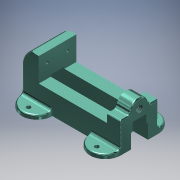
# Autodesk Inventor part: VS-001 (BASE)
Saved by Autodesk Inventor 2017 (Build 210142000, 142)
## iProperties
Created: 2016-11-28
Part Number: VS-001 (BASE)
Material: Iron, Cast
Document SubType Name: Modeling
Designer: OCCC
Mass: 2711.86 g
Surface Area: 697.582 cm^2
Volume: 379.281 cm^3
Density: 7.15 g/cm^3
Appearance: Machined 02
Author: OCCC
Autodesk Inventor part; units mm, degrees
ref_plane "YZ Plane" through (0, 0, 0) normal (1, 0, 0) x (0, 1, 0)
sketch "Sketch1" plane through (0, 0, 0) normal (0, 0, 1) x (1, 0, 0)
  line L0 (0, 0) -> (-184.15, 0)
  line L1 (-184.15, 0) -> (-184.15, 53.975)
  line L2 (-166.8312, 84.1375) -> (-152.4, 84.1375)
  line L3 (-152.4, 84.1375) -> (-152.4, 39.6875)
  line L4 (-152.4, 39.6875) -> (-25.4, 39.6875)
  line L5 (-25.4, 39.6875) -> (-25.4, 55.5625)
  line L6 (-25.4, 55.5625) -> (0, 55.5625)
  line L7 (0, 55.5625) -> (0, 0)
  line L8 (-184.15, 53.975) -> (-149.225, 53.975) construction
  arc A0 (-166.8312, 84.1375) -> (-184.15, 53.975) centre (-149.225, 53.975) ccw
  dimension "d0" = 184.15
  dimension "d1" = 55.5625
  dimension "d4" = 25.4
  dimension "d5" = 15.875
  dimension "d6" = 127
  dimension "d7" = 30.1625
  dimension "d8" = 34.925
  dimension "d9" = 84.1375
  constraints: 18 end point, 7 perpendicular, 2 horizontal, 2 point on circle, 1 centre point, 1 coincident
  measures "d0" distance of L0.start L0.end
  measures "d1" distance of L6.end L0.start
  measures "d4" distance of L5.end L6.end
  measures "d5" distance of L4.end L5.end
  measures "d6" distance of L3.end L4.end
  measures "d7" distance between parallel lines of L2 L8
  measures "d8" distance of L1.end L8.end
  measures "d9" distance between parallel lines of L0 L2
extrude "Extrusion1" add sketch "Sketch1" against normal blind 69.85
sketch "Sketch2" plane through (0, 0, 0) normal (0, 1, 0) x (-1, 0, 0)
  arc A0 (184.15, 0) -> (127, 0) centre (155.575, 0) ccw
  circle A1 centre (155.575, 15.875) radius 3.9688
  line L0 (184.15, 0) -> (127, 0)
  dimension "d12" = 28.575
  dimension "d14" = 7.9375
  dimension "d16" = 57.15
  dimension "d17" = 15.875
  dimension "d18" = 28.575
  constraints: 2 centre point, 2 end point, 2 point on circle, 1 vertical alignment
  measures "d12" radius of A0
  measures "d14" diameter of A1
  measures "d16" distance of L0.start L0.end
  measures "d17" distance from line of L0 A1.centre
  measures "d18" horizontal distance of L0.start A1.centre
extrude "Extrusion2" add sketch "Sketch2" along normal blind 7.9375
ref_plane "Work Plane2" through (0, 0, -34.925) normal (0, 0, 1) x (1, 0, 0)
mirror "Mirror1" about plane through (0, 0, -34.925) normal (0, 0, 1) of "Extrusion2"
ref_plane "Work Plane3" through (-92.075, 0, 0) normal (1, 0, 0) x (0, 0, -1)
mirror "Mirror3" about plane through (-92.075, 0, 0) normal (1, 0, 0) of "Extrusion2", "Mirror1"
sketch "Sketch3" plane through (0, 55.5625, 0) normal (1, 0, 0) x (0, 0, -1)
  arc A0 (52.3152, 0) -> (17.5348, 0) centre (34.925, 1.5875) ccw
  line L0 (0, -55.5625) -> (69.85, -55.5625) projected
  line L1 (69.85, 0) -> (69.85, -47.625) projected
  line L2 (0, 0) -> (69.85, 0) projected
  line L3 (17.5348, 0) -> (52.3152, 0)
  dimension "d28" = 57.15
  dimension "d29" = 34.925
  dimension "d30" = 34.925
  constraints: 2 end point, 2 point on circle, 2 point on line, 1 centre point
  measures "d28" distance from line of L0 A0.centre
  measures "d29" diameter of A0
  measures "d30" distance from line of L1 A0.centre
extrude "Extrusion3" add sketch "Sketch3" against normal blind 25.4
sketch "Sketch4" plane through (0, 7.9375, 0) normal (1, 0, 0) x (0, 0, -1)
  line L0 (34.925, -12.7) -> (34.925, 76.2) construction
  line L1 (69.85, 47.625) -> (69.85, 0) projected
  line L2 (0, -7.9375) -> (69.85, -7.9375) projected
  line L3 (19.0246, -7.9375) -> (19.0246, 19.05)
  line L4 (19.0246, 19.05) -> (22.1996, 19.05)
  line L5 (22.1996, 19.05) -> (22.1996, 34.925)
  line L6 (22.1996, 34.925) -> (47.6504, 34.925)
  line L7 (47.6504, 34.925) -> (47.6504, 19.05)
  line L8 (47.6504, 19.05) -> (50.8254, 19.05)
  line L9 (50.8254, 19.05) -> (50.8254, -7.9375)
  line L10 (19.0246, -7.9375) -> (50.8254, -7.9375)
  line L11 (0, 76.2) -> (69.85, 76.2) projected
  dimension "d33" = 34.925
  dimension "d34" = 12.7254
  dimension "d35" = 15.9004
  dimension "d36" = 25.4508
  dimension "d37" = 31.8008
  dimension "d38" = 26.9875
  dimension "d39" = 42.8625
  dimension "d40" = 88.9
  constraints: 18 end point, 6 perpendicular, 2 collinear, 2 point on line, 2 vertical, 1 midpoint
  measures "d33" distance between parallel lines of L1 L0
  measures "d34" distance between parallel lines of L0 L5
  measures "d35" distance between parallel lines of L9 L0
  measures "d36" distance between parallel lines of L7 L5
  measures "d37" distance between parallel lines of L9 L3
  measures "d38" distance between parallel lines of L2 L8
  measures "d39" distance between parallel lines of L6 L2
  measures "d40" distance of L0.start L0.end
extrude "Extrusion4" cut sketch "Sketch4" against normal through all
fillet "1/4R Fillet" radius 6.35 6 edges at (-155.575, 7.9375, 0) (-28.575, 7.9375, 0) (-12.7, 55.5625, -17.5348) (-12.7, 55.5625, -52.3152) (-28.575, 7.9375, -69.85) (-155.575, 7.9375, -69.85)
fillet "1/8R Fillet" radius 3.175 24 edges at (-184.15, 34.1312, 0) (-184.1091, 10.156, 1.5278) (-155.575, 7.9375, 28.575) (-127.0409, 10.156, 1.5278) (-179.5124, 71.3655, 0) (-0.0409, 10.156, 1.5278) (-28.575, 7.9375, 28.575) (-57.1091, 10.156, 1.5278) (0, 34.925, 0) (-12.7, 55.5625, 0) (0, 56.9938, -15.6097) (0, 74.6125, -34.925) (0, 56.9938, -54.2403) (0, 55.5625, -64.0532) (0, 55.5625, -5.7968) (-0.0409, 10.156, -71.3778) (-28.575, 7.9375, -98.425) (-57.1091, 10.156, -71.3778) (0, 34.925, -69.85) (-184.15, 34.1312, -69.85) (-184.1091, 10.156, -71.3778) (-155.575, 7.9375, -98.425) (-127.0409, 10.156, -71.3778) (-179.5124, 71.3655, -69.85)
hole "5/8-8ACME" at (0, 57.15, -34.925) direction (-1, 0, 0) diameter 12.7 end up to surface thread size "5/8-8 Acme" class "2G" standard "Acme Threads"
hole "(1) 1/4-20UNC-2B" at (-152.4, 65.0875, -53.975) direction (-1, 0, 0) diameter 4.9784 depth 15.875 thread size "1/4-20 UNC" class "2B" standard "ANSI Unified Screw Threads"
hole "(2) 1/4-20UNC-2B" at (-152.4, 65.0875, -15.875) direction (-1, 0, 0) diameter 4.9784 depth 15.875 thread size "1/4-20 UNC" class "2B" standard "ANSI Unified Screw Threads"
body "Solid1"
